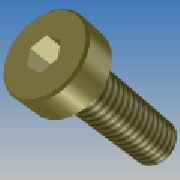
# Autodesk Inventor part: SCREW,LOW SOCKET HD M6x1x20MM
Saved by Autodesk Inventor 2022.4 (Build 264492000, 492)
## iProperties
Category: _
Manager: 606-16872
Created: 2002-03-13
Part Number: SCREW,LOW SOCKET HD M6x1x20MM
Material: Purchased Component, Altered
Description: SCREW,LOW SOCKET HD M6x1x20MM
Document SubType Name: Modeling
Designer: Clint.Matte
Density: 1 g/cm^3
Appearance: Gunmetal
Engr Approved By: P
Checked By: 0000630389
User Status: Released
Mass: 0.825618 g
Surface Area: 7.03265 cm^2
Volume: 0.825618 cm^3
Mfg Approved By: -
Control State: 0
Master: False
Checked Out: False
Shininess: 41.0
Angle Display Precision: 2
Document Length Units: 11269
Document Angle Units: 11279
Document Time Units: 11290
Document Mass Units: 11283
Document Length Units Precision: 3
Document Angle Units Precision: 2
Compacted: True
PTC_WM_ITERATION: 2
PTC_WM_ORGANIZATION_ID: CLWC
PTC_WM_LIFECYCLE: CLWC_CAD_LC
CN_MASS: 0.000826
FIRST_DESCRIPTION: WV
SECOND_DESCRIPTION: _
THIRD_DESCRIPTION: _
CN_SERVICEABLE: _
CL_runCount: 1
FinishProperty: ToBeSet
CN_DESIGNER: -
Density: 0.0
Volumn: 0.0
Area: 0.0
PropertySet Name: Model Information
Subject: 31161518
Keywords: FASTENAL
Revision Number: A
Author: -
Autodesk Inventor part; units mm, degrees
ref_plane "YZ Plane" through (0, 0, 0) normal (1, 0, 0) x (0, 1, 0)
ref_plane "XZ Plane" through (0, 0, 0) normal (0, 1, 0) x (-1, 0, 0)
ref_plane "XY Plane" through (0, 0, 0) normal (0, 0, 1) x (1, 0, 0)
sketch "Sketch1" plane through (0, 0, 0) normal (0, 0, 1) x (1, 0, 0)
  circle A0 centre (0.077, 3.0817) radius 3
  dimension "Diameter" = 6
  constraints: 1 centre point
  measures "Diameter" diameter of A0
extrude "Extrusion1" add sketch "Sketch1" along normal blind 20
sketch "Sketch2" plane through (0.077, 3.0817, 20) normal (0, 0, 1) x (1, 0, 0)
  circle A0 centre (0, 0) radius 3 projected
  circle A1 centre (0, 0) radius 5
  dimension "Head_Diameter" = 10
  constraints: 1 centre point, 1 coincident
  measures "Head_Diameter" diameter of A1
extrude "Extrusion2" add sketch "Sketch2" along normal blind 4 contours A0 | A1
sketch "Sketch3" plane through (0.077, 3.0817, 24) normal (0, 0, 1) x (1, 0, 0)
  circle A0 centre (0, 0) radius 5 projected
  line L0 (0, -2.3094) -> (-2, -1.1547)
  line L1 (-2, -1.1547) -> (-2, 1.1547)
  line L2 (-2, 1.1547) -> (0, 2.3094)
  line L3 (0, 2.3094) -> (2, 1.1547)
  line L4 (2, 1.1547) -> (2, -1.1547)
  line L5 (2, -1.1547) -> (0, -2.3094)
  dimension "Hex_Key_Size" = 4
  constraints: 12 end point, 1 coincident, 11 other
  measures "Hex_Key_Size" distance between parallel lines of L4 L1
extrude "Extrusion3" cut sketch "Sketch3" against normal blind 3.8 contours L0 L1 L2 L3 L4 L5
thread "Thread1" size "M6x1" class "6g" standard "ANSI Metric M Profile" length 18
fillet "Fillet1" radius 0.2 1 edges at (-2.923, 3.0817, 20)
chamfer "Chamfer1" distance 0.25 angle 45 2 edges at (-4.923, 3.0817, 24) (-2.923, 3.0817, 0)
equation "\"d9\" = Thread_Length"
equation "\"d13\" = Chamfer"
equation "\"Thread_Length\" = 18"
equation "\"Chamfer\" = 0.25"
body "Solid1"
